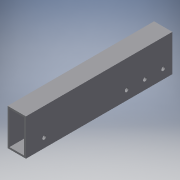
# Autodesk Inventor part: 1x2
Saved by Autodesk Inventor 2018 (Build 220112000, 112)
## iProperties
Created: 2019-01-23
Part Number: 1x2
Material: Generic
Document SubType Name: Modeling
Designer: s-4008082
Density: 1 g/cm^3
Appearance: Default
Mass: 72.9892 g
Surface Area: 585.238 cm^2
Volume: 72.9892 cm^3
Author: s-4008082
Autodesk Inventor part; units mm, degrees
ref_plane "YZ Plane" through (0, 0, 0) normal (1, 0, 0) x (0, 1, 0)
ref_plane "XZ Plane" through (0, 0, 0) normal (0, 1, 0) x (-1, 0, 0)
ref_plane "XY Plane" through (0, 0, 0) normal (0, 0, 1) x (1, 0, 0)
sketch "Sketch1" plane through (0, 0, 0) normal (0, 0, 1) x (1, 0, 0)
  line L0 (0, 0) -> (25.4, 0)
  line L1 (25.4, 0) -> (25.4, 50.8)
  line L2 (25.4, 50.8) -> (0, 50.8)
  line L3 (0, 50.8) -> (0, 0)
  line L4 (22.86, 48.26) -> (2.54, 48.26)
  line L5 (2.54, 48.26) -> (2.54, 2.54)
  line L6 (2.54, 2.54) -> (22.86, 2.54)
  line L7 (22.86, 2.54) -> (22.86, 48.26)
  dimension "d0" = 50.8
  dimension "d1" = 25.4
  dimension "d2" = 2.54
  dimension "d3" = 2.54
  dimension "d4" = 2.54
  dimension "d5" = 2.54
  constraints: 16 end point, 4 parallel, 2 horizontal, 2 perpendicular
  measures "d0" distance of L0.end L1.end
  measures "d1" distance of L1.end L2.end
  measures "d2" distance between parallel lines of L1 L7
  measures "d3" distance between parallel lines of L3 L5
  measures "d4" distance between parallel lines of L0 L6
  measures "d5" distance between parallel lines of L2 L4
extrude "Extrusion1" add sketch "Sketch1" along normal blind 203.2
sketch "Sketch2" plane through (25.4, 0, 0) normal (1, 0, 0) x (0, 0, -1)
  circle A0 centre (-12.7, 12.7) radius 2.5797
  circle A1 centre (-63.5, 12.7) radius 2.5797
  circle A2 centre (-38.1, 12.7) radius 2.5797
  line L0 (0, 2.54) -> (-203.2, 2.54) projected
  line L1 (0, 0) -> (-203.2, 0) projected
  line L2 (0, 0) -> (0, 50.8) projected
  line L3 (-203.2, 0) -> (-203.2, 50.8) projected
  dimension "d8" = 5.1594
  dimension "d10" = 5.1594
  dimension "d11" = 5.1594
  dimension "d12" = 12.7
  dimension "d13" = 12.7
  dimension "d14" = 12.7
  dimension "d16" = 12.7
  dimension "d18" = 38.1
  dimension "d21" = 25.4
  constraints: 3 centre point
  measures "d8" diameter of A2
  measures "d10" diameter of A1
  measures "d11" diameter of A0
  measures "d12" distance from line of L1 A0.centre
  measures "d13" distance from line of L1 A2.centre
  measures "d14" distance from line of L1 A1.centre
  measures "d16" distance from line of L2 A0.centre
  measures "d18" distance from line of L2 A2.centre
  measures "d21" distance of A2.centre A1.centre
extrude "Extrusion2" cut sketch "Sketch2" against normal blind 203.2 contours A0 | A1 | A2
sketch "Sketch3" plane through (25.4, 0, 0) normal (1, 0, 0) x (0, 0, -1)
  circle A0 centre (-138.2776, 12.7) radius 2.5797
  line L0 (-203.2, 0) -> (-203.2, 50.8) projected
  line L1 (0, 0) -> (-203.2, 0) projected
  dimension "d24" = 5.1594
  dimension "d25" = 64.9224
  dimension "d26" = 12.7
  constraints: 1 centre point
  measures "d24" diameter of A0
  measures "d25" distance from line of L0 A0.centre
  measures "d26" distance from line of L1 A0.centre
extrude "Extrusion3" cut sketch "Sketch3" against normal blind 203.2
sketch "Sketch4" plane through (0, 0, 0) normal (-1, 0, 0) x (0, 0, 1)
  circle A0 centre (177.8, 25.4) radius 14.2875
  line L0 (203.2, 50.8) -> (203.2, 0) projected
  line L1 (0, 0) -> (203.2, 0) projected
  dimension "d29" = 28.575
  dimension "d31" = 25.4
  dimension "d32" = 25.4
  constraints: 1 centre point
  measures "d29" diameter of A0
  measures "d31" distance from line of L0 A0.centre
  measures "d32" distance from line of L1 A0.centre
extrude "Extrusion4" cut sketch "Sketch4" against normal blind 25.4
equation "\"d3\" = d2"
equation "\"d4\" = d2"
equation "\"d5\" = d2"
body "Solid1"
